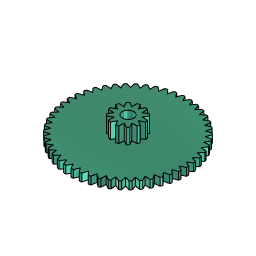
MG996R_Gear_1 v4 (Autodesk Fusion 360 design; units mm, degrees)
Autodesk Fusion 360 part; units mm, degrees
sketch "Sketch1" plane through (0, 0, 0) normal (0, 0, 1) x (1, 0, 0)
  circle A0 centre (0, 0) radius 2
  circle A1 centre (0, 0) radius 7.85
  dimension "d1" = 4
  dimension "d2" = 15.7
  constraint coincident A0.centre A1.centre
  measures "d1" diameter of A0
  measures "d2" diameter of A1
extrude "Extrude1" add sketch "Sketch1" along normal blind 1 contours A0 | A1
extrude "Extrude2" add sketch "Sketch1" along normal blind 3 contours A0
sketch "Sketch2" plane through (0, 0, 3) normal (0, 0, 1) x (-1, 0, 0)
  circle A0 centre (0, 0) radius 2
  circle A1 centre (0, 0) radius 0.75
  dimension "d7" = 1.5
  constraint concentric A0 A1
  measures "d7" diameter of A1
extrude "Extrude3" cut sketch "Sketch2" against normal blind 7 contours A1
sketch "Sketch3" plane through (0, 0, 3) normal (0, 0, 1) x (-1, 0, 0)
  circle A0 centre (0, 0) radius 0.75
  circle A1 centre (0, 0) radius 2
  circle A2 centre (0, 0) radius 2
  line L0 (0.35, -1.9691) -> (0, -1.3629)
  line L1 (0, -1.3629) -> (-0.35, -1.9691)
  dimension "d10" = 0.7
  dimension "d11" = 0.7
  constraint coincident A0.centre A1.centre
  constraint coincident A1 L0.start
  constraint coincident A2 L1.end
  constraint equal L0 L1
  constraint vertical A0.centre L0.end
  constraint equal A1 A2
  measures "d10" distance of L0.start L0.end
  measures "d11" horizontal distance of L0.start L1.end
extrude "Extrude4" cut sketch "Sketch3" against normal blind 2 contours A1 A2 L0 L1 picked at (0, -1.7853)
pattern_circular "C-Pattern1" count 12 over 360 about axis through (0, 0, 3) along (0, 0, -1) of "Extrude4"
sketch "Sketch4" plane through (0, 0, 1) normal (0, 0, 1) x (-1, 0, 0)
  line L0 (-0.6815, -1.8803) -> (-0.6815, -1.1803)
  line L1 (-0.6815, -1.1803) -> (-1.2877, -1.5303)
  line L2 (-1.5303, -1.2877) -> (-1.1803, -0.6815)
  line L3 (-1.1803, -0.6815) -> (-1.8803, -0.6815)
  line L4 (-1.9691, -0.35) -> (-1.3629, 0)
  line L5 (-1.3629, 0) -> (-1.9691, 0.35)
  line L6 (-1.8803, 0.6815) -> (-1.1803, 0.6815)
  line L7 (-1.1803, 0.6815) -> (-1.5303, 1.2877)
  line L8 (-1.2877, 1.5303) -> (-0.6815, 1.1803)
  line L9 (-0.6815, 1.1803) -> (-0.6815, 1.8803)
  line L10 (-0.35, 1.9691) -> (0, 1.3629)
  line L11 (0, 1.3629) -> (0.35, 1.9691)
  line L12 (0.6815, 1.8803) -> (0.6815, 1.1803)
  line L13 (0.6815, 1.1803) -> (1.2877, 1.5303)
  line L14 (1.5303, 1.2877) -> (1.1803, 0.6815)
  line L15 (1.1803, 0.6815) -> (1.8803, 0.6815)
  line L16 (1.9691, 0.35) -> (1.3629, 0)
  line L17 (1.3629, 0) -> (1.9691, -0.35)
  line L18 (1.8803, -0.6815) -> (1.1803, -0.6815)
  line L19 (1.1803, -0.6815) -> (1.5303, -1.2877)
  line L20 (1.2877, -1.5303) -> (0.6815, -1.1803)
  line L21 (0.6815, -1.1803) -> (0.6815, -1.8803)
  line L22 (0.35, -1.9691) -> (0, -1.3629)
  line L23 (0, -1.3629) -> (-0.35, -1.9691)
  circle A0 centre (0, 0) radius 7.85
  circle A1 centre (0, 0) radius 7.85
  line L24 (0.35, -7.8422) -> (0, -7.236)
  line L25 (0, -7.236) -> (-0.35, -7.8422)
  arc A2 (-0.6815, -1.8803) -> (-0.35, -1.9691) centre (0, 0) ccw
  arc A3 (-1.5303, -1.2877) -> (-1.2877, -1.5303) centre (0, 0) ccw
  arc A4 (-1.9691, -0.35) -> (-1.8803, -0.6815) centre (0, 0) ccw
  arc A5 (-1.8803, 0.6815) -> (-1.9691, 0.35) centre (0, 0) ccw
  arc A6 (-1.2877, 1.5303) -> (-1.5303, 1.2877) centre (0, 0) ccw
  arc A7 (-0.35, 1.9691) -> (-0.6815, 1.8803) centre (0, 0) ccw
  arc A8 (0.6815, 1.8803) -> (0.35, 1.9691) centre (0, 0) ccw
  arc A9 (1.5303, 1.2877) -> (1.2877, 1.5303) centre (0, 0) ccw
  arc A10 (1.9691, 0.35) -> (1.8803, 0.6815) centre (0, 0) ccw
  arc A11 (1.8803, -0.6815) -> (1.9691, -0.35) centre (0, 0) ccw
  arc A12 (1.2877, -1.5303) -> (1.5303, -1.2877) centre (0, 0) ccw
  arc A13 (0.35, -1.9691) -> (0.6815, -1.8803) centre (0, 0) ccw
  dimension "d16" = 0.7
  dimension "d17" = 0.7
  constraint coincident A0.centre A1.centre
  constraint coincident A1 L24.start
  constraint coincident A1 L25.end
  constraint equal L24 L25
  constraint vertical A0.centre L24.end
  constraint equal A0 A1
  measures "d16" distance of L24.start L24.end
  measures "d17" distance of L24.start L25.end
extrude "Extrude5" cut sketch "Sketch4" against normal blind 1.3 contours A0 A1 L24 L25 picked at (0, -7.6447)
pattern_circular "C-Pattern2" count 50 over 360 about axis through (0, 0, 1.75) along (0, 0, 1) of "Extrude5"
